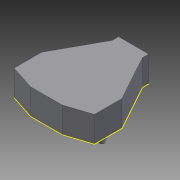
# Autodesk Inventor part: Inkjet
Saved by Autodesk Inventor 2015 (Build 190159000, 159)
## iProperties
Created: 2015-06-18
Part Number: Inkjet
Material: Generic
Document SubType Name: Modeling
Designer: Oliver
Density: 1 g/cm^3
Appearance: Default
Author: Oliver
Autodesk Inventor part; units mm, degrees
ref_plane "YZ Plane" through (0, 0, 0) normal (1, 0, 0) x (0, 1, 0)
ref_plane "XZ Plane" through (0, 0, 0) normal (0, 1, 0) x (-1, 0, 0)
ref_plane "XY Plane" through (0, 0, 0) normal (0, 0, 1) x (1, 0, 0)
sketch "Sketch1" plane through (0, 0, 0) normal (0, 0, 1) x (1, 0, 0)
  line L0 (-5, -2.5) -> (5, -2.5)
  line L1 (5, -2.5) -> (12.675, 0)
  line L2 (-5, -2.5) -> (-12.675, 0)
  line L3 (12.675, 0) -> (-12.675, 0) construction
  line L4 (12.675, 0) -> (12.675, 8.7)
  line L5 (-12.675, 0) -> (-12.675, 8.7)
  line L6 (-12.675, 8.7) -> (-4.75, 23.1)
  line L7 (-4.75, 23.1) -> (-4.75, 25.1)
  line L8 (-4.75, 25.1) -> (4.75, 25.1)
  line L9 (4.75, 25.1) -> (4.75, 23.1)
  line L10 (4.75, 23.1) -> (12.675, 8.7)
  line L11 (0, -8.02) -> (0, 30.62) projected
  line L12 (0, 25.1) -> (0, -2.5)
  point P0 (0, 0)
  point P1 (0, 0)
  dimension "d0" = 10
  dimension "d1" = 25.35
  dimension "d2" = 2.5
  dimension "d3" = 8.7
  dimension "d4" = 27.6
  dimension "d6" = 2
  dimension "d7" = 9.5
  constraints: 24 end point, 4 equal length, 4 vertical, 3 horizontal, 3 midpoint, 2 point on line, 1 coincident
  measures "d0" distance of L0.start L0.end
  measures "d1" distance of L1.end L2.end
  measures "d2" distance between parallel lines of L3 L0
  measures "d3" distance of L1.end L4.end
  measures "d4" distance between parallel lines of L0 L8
  measures "d6" distance of L8.end L9.end
  measures "d7" distance of L7.end L8.end
extrude "Body" add sketch "Sketch1" along normal blind 8.1 contours L11 L8 L9 L10 L4 L1 L0
sketch "Sketch5" plane through (0, 0, 0) normal (0, 0, -1) x (-1, 0, 0)
  circle A0 centre (-10.8, 4.25) radius 1.25
  line L0 (-10.8, 4.25) -> (0, 4.25) construction
  line L1 (0, 25.1) -> (0, -2.5) projected
  line L2 (0, -2.5) -> (-5, -2.5) projected
  point P0 (0, 0)
  dimension "d26" = 2.5
  dimension "d27" = 10.8
  dimension "d28" = 6.75
  constraints: 2 end point, 1 centre point, 1 horizontal, 1 point on line
  measures "d26" diameter of A0
  measures "d27" distance of L0.start L0.end
  measures "d28" distance between parallel lines of L2 L0
extrude "PinCylinder" add sketch "Sketch5" along normal blind 1
ref_plane "Work Plane3" through (10.8, 4.25, -2.5) normal (0, 0, -1) x (-1, 0, 0)
sketch "Sketch6" plane through (10.8, 4.25, -2.5) normal (0, 0, -1) x (-1, 0, 0)
  circle A0 centre (0, 0) radius 1.25 projected
  circle A1 centre (0, 0) radius 0.75
  point P0 (10.8, -4.25)
  dimension "d32" = 1.5
  constraints: 1 centre point
  measures "d32" diameter of A1
loft "Loft2" add profiles "Sketch6" section 1 edges at (12.05, 4.25, -1) contours A1
sketch "Sketch7" plane through (0, 0, 0) normal (0, 0, -1) x (-1, 0, 0)
  line L0 (0, -0.7) -> (-4.15, -0.7)
  line L1 (-4.15, -0.7) -> (-4.15, 24.1)
  line L2 (0, -2.5) -> (-5, -2.5) projected
  line L3 (0, 25.1) -> (0, -2.5) projected
  line L4 (-4.15, 24.1) -> (0, 24.1)
  point P0 (0, 0)
  dimension "d37" = 4.15
  dimension "d38" = 24.8
  dimension "d39" = 1.8
  constraints: 6 end point, 2 horizontal, 2 point on line, 1 perpendicular
  measures "d37" distance of L0.start L0.end
  measures "d38" distance of L0.end L1.end
  measures "d39" distance between parallel lines of L2 L0
extrude "MiddleCutout" cut sketch "Sketch7" against normal blind 1
mirror "Mirror1" about plane through (0, 25.1, 0) normal (-1, 0, 0)
sketch "Sketch8" plane through (0, 0, 0) normal (0, 0, -1) x (-1, 0, 0)
  line L0 (-4.75, 25.1) -> (4.75, 25.1) projected
  line L1 (-4.75, 23.1) -> (-4.75, 25.1) projected
  line L2 (-12.675, 8.7) -> (-4.75, 23.1) projected
  line L3 (-12.675, 0) -> (-12.675, 8.7) projected
  line L4 (-5, -2.5) -> (-12.675, 0) projected
  line L5 (-5, -2.5) -> (5, -2.5) projected
  line L6 (5, -2.5) -> (12.675, 0) projected
  line L7 (12.675, 0) -> (12.675, 8.7) projected
  line L8 (12.675, 8.7) -> (4.75, 23.1) projected
  line L9 (4.75, 23.1) -> (4.75, 25.1) projected
  circle A0 centre (10.8, 4.25) radius 1.25 projected
  line L10 (-4.15, 24.1) -> (4.15, 24.1) projected
  line L11 (4.15, -0.7) -> (4.15, 24.1) projected
  line L12 (4.15, -0.7) -> (-4.15, -0.7) projected
  line L13 (-4.15, -0.7) -> (-4.15, 24.1) projected
  circle A1 centre (-10.8, 4.25) radius 1.25 projected
  point P0 (0, 0)
body "Solid3"
